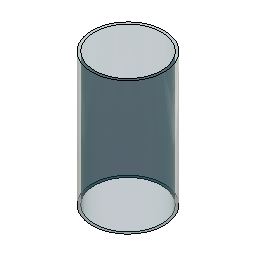
Glass_Chamber (Autodesk Fusion 360 design; units mm, degrees)
Autodesk Fusion 360 part; units mm, degrees
sketch "Sketch2" plane through (0, 0, 0) normal (0, 1, 0) x (1, 0, 0)
  circle A0 centre (0, 0) radius 19
  dimension "d3" = 38
  constraint coincident A0.centre origin
  measures "d3" diameter of A0
extrude "Extrude1" add sketch "Sketch2" along normal blind 70
sketch "Sketch4" plane through (0, 70, 0) normal (0, 1, 0) x (-1, 0, 0)
  circle A0 centre (0, 0) radius 19
  circle A1 centre (0, 0) radius 17.6
  dimension "d11" = 35.2
  constraint coincident A0.centre A1.centre
  measures "d11" diameter of A1
extrude "Extrude4" cut sketch "Sketch4" against normal through all contours A1
